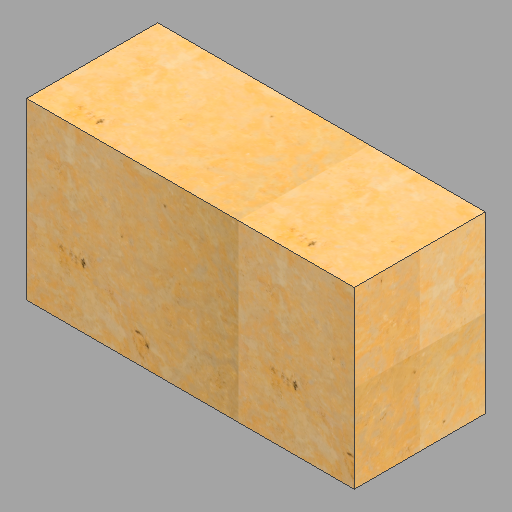
# Autodesk Inventor part: 24x18x80lf
Saved by Autodesk Inventor 2023 (Build 270158000, 158)
## iProperties
RuleStatus: InUse
Created: 2022-04-19
Part Number: 24x18x80lf
Material: Granite, Cut, Polished
Document SubType Name: Modeling
Designer: awelt
Mass: 860124 g
Surface Area: 29961.2 cm^2
Volume: 318565 cm^3
Density: 2.7 g/cm^3
Appearance: Amber Select
AfterDocOpen0: Convert in3 volume to ft3
AfterDocSave0: Convert in3 volume to ft3
AfterDocSave1: Convert in3 volume to ft3
AfterAnyUserParamChange0: Convert in3 volume to ft3
in3 to ft3: 11.25
TEST: 11.25
Author: awelt
Autodesk Inventor part; units mm, degrees
ref_plane "YZ Plane" through (0, 0, 0) normal (1, 0, 0) x (0, 1, 0)
ref_plane "XZ Plane" through (0, 0, 0) normal (0, 1, 0) x (-1, 0, 0)
ref_plane "XY Plane" through (0, 0, 0) normal (0, 0, 1) x (1, 0, 0)
sketch "Sketch1" plane through (0, 0, 0) normal (1, 0, 0) x (0, 1, 0)
  line L0 (0, 0) -> (609.6, 0)
  line L1 (609.6, 0) -> (609.6, 457.2)
  line L2 (609.6, 457.2) -> (0, 457.2)
  line L3 (0, 457.2) -> (0, 0)
  dimension "d0" = 609.6
  dimension "d1" = 457.2
  constraints: 8 end point, 2 parallel, 1 horizontal, 1 perpendicular
  measures "d0" distance of L2.end L1.end
  measures "d1" distance of L1.end L0.end
extrude "Extrusion1" add sketch "Sketch1" along normal blind 1143
body "Solid1"
